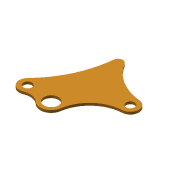
# Autodesk Inventor part: 3136 1133 85
Saved by Autodesk Inventor 2022 Beta2 (Build 260130000, 130) ContinuousBuild 0
## iProperties
Shininess: 64.0
Length Units: 11269
Angle Units: 11279
Time Units: 11290
Mass Units: 11283
Length Display Precision: 3
Angle Display Precision: 2
Compacted: True
Part Number: 3136 1133 85
Document SubType Name: Modeling
Created: 2003-04-13
Designer: Uffe Bak
Material: Steel, Mild
Density: 7.86 g/cm^3
Appearance: Brokk-Gul
Density: 0.0
Volumn: 0.0
Area: 0.0
PropertySet Name: Model Information
Control State: 0
Master: False
Checked Out: False
Author: Uffe Bak
Autodesk Inventor part; units mm, degrees
ref_plane "YZ Plane" through (0, 0, 0) normal (1, 0, 0) x (0, 1, 0)
ref_plane "XZ Plane" through (0, 0, 0) normal (0, 1, 0) x (-1, 0, 0)
ref_plane "XY Plane" through (0, 0, 0) normal (0, 0, 1) x (1, 0, 0)
sketch "Sketch1" plane through (0, 0, 0) normal (0, 0, 1) x (0, 1, 0)
  circle A0 centre (103.8572, -128.4288) radius 17.5
  circle A1 centre (-46.1428, 47.5712) radius 30
  circle A2 centre (-36.5428, 154.0712) radius 17.5
  arc A3 (-12.2627, 179.2798) -> (-68.6436, 140.1233) centre (-36.5428, 154.0712) ccw
  arc A4 (-79.1765, 78.1289) -> (-52.7383, 3.0571) centre (-46.1428, 47.5712) ccw
  arc A5 (68.91, -130.351) -> (138.7018, -131.7234) centre (103.8572, -128.4288) ccw
  arc A6 (239.3875, 30.5679) -> (230.7678, 67.4797) centre (228.8572, 47.5712) ccw
  arc A7 (-79.1765, 78.1289) -> (-68.6436, 140.1233) centre (-121.4095, 117.1964) ccw
  arc A8 (68.91, -130.351) -> (-52.7383, 3.0571) centre (-73.6667, -138.1931) ccw
  arc A9 (239.3875, 30.5679) -> (138.7018, -131.7234) centre (352.4092, -151.9293) ccw
  arc A10 (-12.2627, 179.2798) -> (230.7678, 67.4797) centre (269.5808, 471.9005) ccw
  dimension "d0" = 106.5
  dimension "d1" = 176
  dimension "d2" = 150
  dimension "d3" = 9.6
  dimension "d4" = 275
  dimension "d5" = 60
  dimension "d6" = 35
  dimension "d7" = 35
  dimension "d8" = 35
  dimension "d9" = 35
  dimension "d10" = 45
  dimension "d11" = 20
  constraints: 22 point on circle, 11 centre point, 8 tangent, 3 coincident, 3 concentric, 1 horizontal alignment
  measures "d0" vertical distance of A2.centre A1.centre
  measures "d1" vertical distance of A0.centre A1.centre
  measures "d2" horizontal distance of A0.centre A1.centre
  measures "d3" horizontal distance of A2.centre A1.centre
  measures "d4" distance of A6.centre A1.centre
  measures "d5" diameter of A1
  measures "d6" diameter of A0
  measures "d7" diameter of A2
  measures "d8" radius of A5
  measures "d9" radius of A3
  measures "d10" radius of A4
  measures "d11" radius of A6
extrude "Extrusion1" add sketch "Sketch1" along normal blind 10
body "Solid1"
